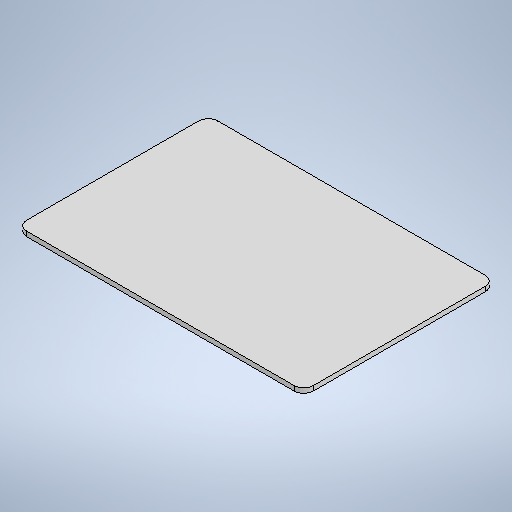
# Autodesk Inventor part: MSC 900.9 base frame transverse
Saved by Autodesk Inventor 2025 (Build 290162010, 162A)
## iProperties
Created: 2024-06-25
Part Number: MSC 900.9 base frame transverse
Material: Stainless Steel
Document SubType Name: Sheet Metal
Designer: DELL
Stock Number: МОО 908 крепление поперечного столба
Density: 8 g/cm^3
Sheet Metal Rule: AISI304 3mm Die 32
Appearance: Default
Mass: 517.658 g
Surface Area: 449.073 cm^2
Volume: 64.7073 cm^3
Flat Pattern Width: 12 cm
Flat Pattern Length: 18 cm
Flat Pattern Area: 216 cm^2
Sheet Metal Width: 120,000 mm
Sheet Metal Length: 180,000 mm
Sheet Metal Area: 21600,000 mm^2
Author: admin
Autodesk Inventor part; units mm, degrees
ref_plane "YZ Plane" through (0, 0, 0) normal (1, 0, 0) x (0, 1, 0)
ref_plane "XZ Plane" through (0, 0, 0) normal (0, 1, 0) x (-1, 0, 0)
ref_plane "XY Plane" through (0, 0, 0) normal (0, 0, 1) x (1, 0, 0)
sketch3d "3D Sketch1"
sketch "Sketch1" plane through (0, 0, 0) normal (0, 0, 1) x (1, 0, 0)
  line L0 (-48, 60) -> (48, 60)
  line L1 (48, 60) -> (48, -60) construction
  line L2 (48, -60) -> (-48, -60)
  line L3 (-48, -60) -> (-48, 60) construction
  line L4 (-48, 60) -> (48, -60) construction
  line L5 (48, 60) -> (-48, -60) construction
  line L6 (48, -60) -> (90, -60)
  line L7 (90, -60) -> (90, 60)
  line L8 (90, 60) -> (48, 60)
  line L9 (-48, -60) -> (-90, -60)
  line L10 (-90, -60) -> (-90, 60)
  line L11 (-90, 60) -> (-48, 60)
  circle A0 centre (70, -45) radius 8.5
  circle A1 centre (70, 45) radius 8.5
  circle A2 centre (-70, -45) radius 8.5
  circle A3 centre (-70, 45) radius 8.5
  line L12 (0, -60) -> (0, 60) construction
  line L13 (90, 0) -> (-90, 0) construction
  point P0 (0, 0)
  dimension "d30" = 120
  dimension "d34" = 180
  dimension "d35" = 17
  dimension "d36" = 20
  dimension "d37" = 15
  measures "d30" distance of L2.end L0.start
  measures "d34" distance between parallel lines of L10 L7
  measures "d35" diameter of A0
  measures "d36" distance from line of L7 A0.centre
  measures "d37" distance from line of L6 A0.centre
extrude "Plate1" add sketch "Sketch1" along normal blind 3 contours L0 L8 L7 L6 L2 L9 L10 L11 | A0 | A1 | A2 | A3
fillet "Corner Round1" radius 6 4 edges at (90, 60, 1.5) (-90, 60, 1.5) (-90, -60, 1.5) (90, -60, 1.5)
equation "\"d6\" = Thickness"
equation "\"BendReliefWidth\" = Thickness"
equation "\"BendReliefDepth\" = 0.5 * Thickness"
equation "\"CornerReliefSize\" = 4 * Thickness"
equation "\"MinimumRemnant\" = 2 * Thickness"
equation "\"TransitionRadius\" = BendRadius"
equation "\"JacobiRadiusSize\" = BendRadius"
equation "\"GapSize\" = Thickness"
equation "\"Thickness\" = 3"
equation "\"BendRadius\" = 5"
body "Solid1"
